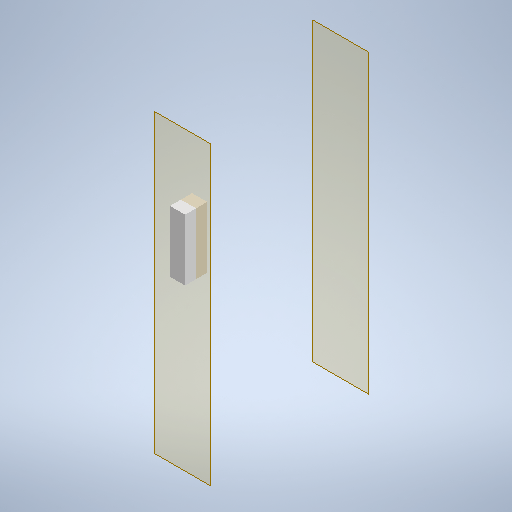
# Autodesk Inventor part: Forward_Motor
Saved by Autodesk Inventor 2027.1 (Build 311270010, 270A)
## iProperties
Created: 2026-09-09
Part Number: Forward_Motor
Material: Generic
Document SubType Name: Modeling
Designer: PWYNNE
Density: 1 g/cm^3
Appearance: Default
Author: PWYNNE
Autodesk Inventor part; units mm, degrees
ref_plane "YZ Plane" through (0, 0, 0) normal (1, 0, 0) x (0, 1, 0)
ref_plane "XZ Plane" through (0, 0, 0) normal (0, 1, 0) x (-1, 0, 0)
ref_plane "XY Plane" through (0, 0, 0) normal (0, 0, 1) x (1, 0, 0)
ref_plane "Work Plane1" through (0, 0, 0) normal (0, 0, 1) x (1, 0, 0)
sketch "Sketch1" plane through (0, 0, 0) normal (0, 0, 1) x (1, 0, 0)
  spline S0 degree 4 poles (136.4096, -125) (139.6804, -111.084) (140.6019, -106.6446) (147.2484, -69.4618) (151.9852, -34.9807) (155.6939, -5.1459) (158.1523, 25.1064) (160.0046, 50.848) (160.2406, 83.7876) (159.6363, 97.5873) (158.2793, 114.9771) (156.6846, 128.0825) (153.6773, 144.318) (151.4216, 151.644) (149.4922, 159.0693) (145.0308, 168.1053) (143.9788, 170.4431) (136.2095, 177.978) (130.6438, 170.533) (129.6208, 167.9907) (126.7812, 158.9537) (125.8674, 151.603) (124.8903, 144.2235) (123.8233, 127.9976) (123.6075, 114.9282) (123.6573, 97.5542) (124.0113, 83.7731) (125.0032, 50.8672) (126.2753, 25.1375) (128.0569, -5.0814) (129.9494, -34.9258) (132.0407, -69.3429) (134.8174, -106.563) (134.7864, -111.0637) (136.3435, -125) knots 0 0 0 0 0 0.079222 0.116044 0.155717 0.19533 0.234892 0.271531 0.305271 0.336139 0.364181 0.390261 0.414415 0.436733 0.455834 0.474841 0.493268 0.510208 0.528357 0.546554 0.565216 0.587182 0.611089 0.637002 0.664944 0.695772 0.729497 0.766123 0.80565 0.845185 0.884726 0.921374 1 1 1 1 1 projected
  line L0 (123.6506, 217.3206) -> (123.6506, 0)
  line L1 (123.6506, 193.5367) -> (75.8602, 193.5367)
  line L2 (75.8602, 193.5367) -> (75.8602, 0)
  line L3 (75.8602, 0) -> (123.6506, 0)
  line L4 (123.6506, 0) -> (123.6506, 193.5367)
  point P0 (0, 0)
  point P1 (123.6506, 108.6603)
  constraints: 10 end point, 2 parallel, 1 horizontal, 1 midpoint, 1 perpendicular, 1 point on line, 1 vertical, 1 other
ref_plane "Work Plane2" through (0, 0, 500) normal (0, 0, 1) x (1, 0, 0)
extrude "Extrusion1" add sketch "Sketch1" along normal mid plane 70 from surface at 500
body "Solid1"
